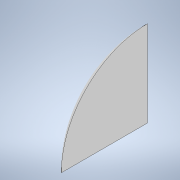
# Autodesk Inventor part: 3DPrintShapeCornerSimplified
Saved by Autodesk Inventor 2022 (Build 260153000, 153)
## iProperties
Created: 2022-04-20
Part Number: 3DPrintShapeCornerSimplified
Material: Generic
Document SubType Name: Modeling
Designer: Bruger
Density: 1 g/cm^3
Appearance: Default
Author: Bruger
Autodesk Inventor part; units mm, degrees
ref_plane "YZ Plane" through (0, 0, 0) normal (1, 0, 0) x (0, 1, 0)
ref_plane "XZ Plane" through (0, 0, 0) normal (0, 1, 0) x (-1, 0, 0)
ref_plane "XY Plane" through (0, 0, 0) normal (0, 0, 1) x (1, 0, 0)
sketch "Sketch1" plane through (0, 0, 0) normal (0, 1, 0) x (-1, 0, 0)
  line L0 (0, 0) -> (0, -150)
  line L1 (0, -150) -> (50, -150)
  line L2 (0, 0) -> (50, -44.9152) construction
  line L3 (50, -44.9152) -> (50, -150) construction
  spline S0 degree 2 poles (0, 0) (50, -44.9152) (50, -150) knots 1 1 1 2 2 2
  dimension "d0" = 150
  dimension "d2" = 50
  constraints: 4 end point, 1 horizontal, 1 vertical, 3 other
  measures "d0" distance of L0.start L0.end
  measures "d2" distance of L0.end L1.end
revolve "Revolution1" add sketch "Sketch1" angle 90 about axis through (0, 0, -150) along (-1, 0, 0)
body "Solid1"
